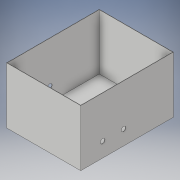
# Autodesk Inventor part: 563-AU1028MG-PE4312
Saved by Autodesk Inventor 2018 (Build 220112000, 112)
## iProperties
Created: 2018-04-30
Part Number: 563-AU1028MG-PE4312
Material: Generic
Document SubType Name: Modeling
Designer: bbramman
Density: 1 g/cm^3
Appearance: Default
Author: bbramman
Autodesk Inventor part; units mm, degrees
ref_plane "YZ Plane" through (0, 0, 0) normal (1, 0, 0) x (0, 1, 0)
ref_plane "XZ Plane" through (0, 0, 0) normal (0, 1, 0) x (-1, 0, 0)
ref_plane "XY Plane" through (0, 0, 0) normal (0, 0, 1) x (1, 0, 0)
sketch "Sketch1" plane through (0, 0, 0) normal (0, 1, 0) x (-1, 0, 0)
  line L0 (-50.8, 63.5) -> (50.8, 63.5)
  line L1 (50.8, 63.5) -> (50.8, -63.5)
  line L2 (50.8, -63.5) -> (-50.8, -63.5)
  line L3 (-50.8, -63.5) -> (-50.8, 63.5)
  line L4 (-50.8, 63.5) -> (50.8, -63.5) construction
  line L5 (50.8, 63.5) -> (-50.8, -63.5) construction
  point P0 (0, 0)
  dimension "d0" = 101.6
  dimension "d1" = 127
  constraints: 12 end point, 2 midpoint, 2 parallel, 1 horizontal, 1 perpendicular
  measures "d0" distance of L1.end L2.end
  measures "d1" distance of L0.end L1.end
extrude "Extrusion1" add sketch "Sketch1" along normal blind 1.016
sketch "Sketch2" plane through (0, 1.016, 0) normal (0, 1, 0) x (1, 0, 0)
  line L0 (50.8, 63.5) -> (-50.8, 63.5) projected
  line L1 (50.8, -63.5) -> (-50.8, -63.5)
  line L2 (-50.8, -63.5) -> (-50.8, 63.5)
  line L3 (-50.8, 63.5) -> (50.8, 63.5)
  line L4 (50.8, 63.5) -> (50.8, -63.5)
  line L5 (50.8, -63.5) -> (-50.8, 63.5) construction
  line L6 (-50.8, -63.5) -> (50.8, 63.5) construction
  line L7 (50.292, -62.992) -> (-50.292, -62.992)
  line L8 (-50.292, -62.992) -> (-50.292, 62.992)
  line L9 (-50.292, 62.992) -> (50.292, 62.992)
  line L10 (50.292, 62.992) -> (50.292, -62.992)
  line L11 (50.292, -62.992) -> (-50.292, 62.992) construction
  line L12 (-50.292, -62.992) -> (50.292, 62.992) construction
  point P0 (0, 0)
  dimension "d4" = 100.584
  dimension "d5" = 125.984
  constraints: 24 end point, 4 midpoint, 4 parallel, 2 horizontal, 2 perpendicular
  measures "d4" distance of L8.end L9.end
  measures "d5" distance of L7.end L8.end
extrude "Extrusion2" add sketch "Sketch2" along normal blind 76.2
sketch "Sketch3" plane through (0, 1.016, 0) normal (0, 1, 0) x (1, 0, 0)
  line L0 (0, 0) -> (0, -25.4)
  line L1 (0, -25.4) -> (0, 25.4)
  circle A0 centre (0, -25.4) radius 2.0828
  circle A1 centre (0, 25.4) radius 2.0828
  dimension "d8" = 25.4
  dimension "d9" = 50.8
  dimension "d10" = 4.1656
  dimension "d11" = 4.1656
  constraints: 4 end point, 2 centre point, 2 coincident, 1 point on line, 1 vertical
  measures "d8" distance of L0.start L0.end
  measures "d9" distance of L0.end L1.end
  measures "d10" diameter of A0
  measures "d11" diameter of A1
extrude "Extrusion3" cut sketch "Sketch3" against normal through all
sketch "Sketch4" plane through (0, 1.016, 0) normal (0, 1, 0) x (1, 0, 0)
  line L0 (24.4983, -44.5008) -> (-24.4983, -44.5008)
  line L1 (-24.4983, 44.5008) -> (24.4983, 44.5008)
  line L2 (24.4983, 44.5008) -> (24.4983, -44.5008)
  line L3 (24.4983, -44.5008) -> (-24.4983, 44.5008) construction
  line L4 (-24.4983, -44.5008) -> (24.4983, 44.5008) construction
  line L5 (21.8694, -44.5008) -> (-21.8694, -44.5008)
  line L6 (-21.8694, 44.5008) -> (21.8694, 44.5008)
  line L7 (21.8694, -44.5008) -> (-21.8694, 44.5008) construction
  line L8 (-21.8694, -44.5008) -> (21.8694, 44.5008) construction
  line L9 (24.4983, 44.5008) -> (-24.4983, 44.5008)
  line L10 (-24.4983, 44.5008) -> (-24.4983, -24.511)
  line L11 (24.4983, -24.511) -> (24.4983, 44.5008)
  line L12 (-21.8694, -44.5008) -> (-18.6944, -44.5008)
  line L13 (21.8694, -44.5008) -> (18.6944, -44.5008)
  line L14 (24.4983, 44.5008) -> (21.3233, 44.5008)
  line L15 (24.4983, 41.3258) -> (24.4983, 44.5008)
  line L16 (-24.4983, 44.5008) -> (-21.3233, 44.5008)
  line L17 (-24.4983, 41.3258) -> (-24.4983, 44.5008)
  circle A0 centre (-18.6944, -41.3258) radius 1.4224
  circle A1 centre (-21.3233, 41.3258) radius 1.4224
  circle A2 centre (21.3233, 41.3258) radius 1.4224
  circle A3 centre (18.6944, -41.3258) radius 1.4224
  point P0 (0, 0)
  dimension "d14" = 48.9966
  dimension "d15" = 89.0016
  dimension "d16" = 43.7388
  dimension "d17" = 89.0016
  dimension "d18" = 69.0118
  dimension "d27" = 2.8448
  dimension "d28" = 2.8448
  dimension "d29" = 2.8448
  dimension "d30" = 2.8448
  constraints: 36 end point, 7 horizontal, 4 centre point, 4 midpoint, 3 parallel, 1 perpendicular
  measures "d14" distance of L1.start L1.end
  measures "d15" distance of L0.end L1.start
  measures "d16" distance of L6.start L6.end
  measures "d17" distance of L5.end L6.start
  measures "d18" distance of L10.end L9.end
  measures "d27" diameter of A0
  measures "d28" diameter of A1
  measures "d29" diameter of A2
  measures "d30" diameter of A3
extrude "Extrusion4" cut sketch "Sketch4" against normal through all
sketch "Sketch5" plane through (0, 1.016, 0) normal (0, 1, 0) x (1, 0, 0)
  line L0 (9.9949, -32.9946) -> (-9.9949, -32.9946)
  line L1 (-9.9949, 32.9946) -> (9.9949, 32.9946)
  line L2 (9.9949, 32.9946) -> (9.9949, -32.9946)
  line L3 (9.9949, -32.9946) -> (-9.9949, 32.9946) construction
  line L4 (-9.9949, -32.9946) -> (9.9949, 32.9946) construction
  circle A0 centre (-9.9949, -32.9946) radius 1.4224
  circle A1 centre (9.9949, -32.9946) radius 1.4224
  circle A2 centre (9.9949, 32.9946) radius 1.4224
  circle A3 centre (-9.9949, 32.9946) radius 1.4224
  point P0 (0, 0)
  dimension "d33" = 19.9898
  dimension "d34" = 65.9892
  dimension "d35" = 2.8448
  dimension "d36" = 2.8448
  dimension "d37" = 2.8448
  dimension "d38" = 2.8448
  constraints: 10 end point, 4 centre point, 4 coincident, 2 midpoint, 1 horizontal, 1 parallel
  measures "d33" distance of L1.start L1.end
  measures "d34" distance of L0.end L1.start
  measures "d35" diameter of A0
  measures "d36" diameter of A1
  measures "d37" diameter of A2
  measures "d38" diameter of A3
extrude "Extrusion5" cut sketch "Sketch5" against normal through all
sketch "Sketch6" plane through (-50.292, 1.016, 62.992) normal (1, 0, 0) x (0, 0, -1)
  line L0 (0, 0) -> (0, 76.2) projected
  line L1 (0, 19.05) -> (18.4912, 19.05)
  line L2 (0, 19.05) -> (18.4912, 19.05) construction
  line L3 (18.4912, 19.05) -> (29.6164, 19.05)
  line L4 (29.6164, 19.05) -> (58.1914, 19.05)
  circle A0 centre (29.6164, 19.05) radius 3.175
  circle A1 centre (58.1914, 19.05) radius 3.175
  point P0 (62.992, -1.016)
  dimension "d41" = 18.4912
  dimension "d42" = 0
  dimension "d43" = 11.1252
  dimension "d44" = 28.575
  dimension "d45" = 180
  dimension "d46" = 6.35
  dimension "d47" = 6.35
  constraints: 8 end point, 2 centre point, 2 coincident, 2 collinear, 2 horizontal, 1 perpendicular, 1 point on line
  measures "d41" distance of L1.start L1.end
  measures "d42" distance between parallel lines of L1 L2
  measures "d43" distance of L2.end L3.end
  measures "d44" distance of L3.end L4.end
  measures "d45" angle of L4 L3
  measures "d46" diameter of A0
  measures "d47" diameter of A1
extrude "Extrusion6" cut sketch "Sketch6" against normal through all
sketch "Sketch7" plane through (50.292, 1.016, -62.992) normal (-1, 0, 0) x (0, 0, 1)
  line L0 (125.984, 0) -> (125.984, 76.2) projected
  line L1 (125.984, 19.05) -> (107.4928, 19.05)
  line L2 (125.984, 19.05) -> (144.4752, 19.05) construction
  line L3 (107.4928, 19.05) -> (96.3676, 19.05)
  line L4 (96.3676, 19.05) -> (67.7926, 19.05)
  circle A0 centre (67.7926, 19.05) radius 3.175
  circle A1 centre (96.3676, 19.05) radius 3.175
  point P0 (62.992, -1.016)
  dimension "d50" = 18.4912
  dimension "d51" = 180
  dimension "d52" = 11.1252
  dimension "d53" = 28.575
  dimension "d54" = 180
  dimension "d55" = 6.35
  dimension "d56" = 6.35
  constraints: 8 end point, 2 centre point, 2 coincident, 2 collinear, 2 point on line, 1 horizontal, 1 perpendicular
  measures "d50" distance of L1.start L1.end
  measures "d51" angle of L1 L2
  measures "d52" distance of L1.end L3.end
  measures "d53" distance of L3.end L4.end
  measures "d54" angle of L4 L3
  measures "d55" diameter of A0
  measures "d56" diameter of A1
extrude "Extrusion7" cut sketch "Sketch7" against normal through all
body "Solid1"
